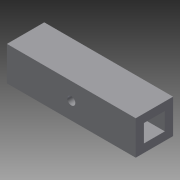
# Autodesk Inventor part: Truc Lumiere
Saved by Autodesk Inventor 2014 SP2 (Build 180246200, 246)
## iProperties
Created: 2014-11-04
Part Number: Truc Lumiere
Material: Générique
Document SubType Name: Modeling
Designer: sd
Density: 1 g/cm^3
Appearance: Par défaut
Author: sd
Autodesk Inventor part; units mm, degrees
ref_plane "YZ Plane" through (0, 0, 0) normal (1, 0, 0) x (0, 1, 0)
ref_plane "XZ Plane" through (0, 0, 0) normal (0, 1, 0) x (-1, 0, 0)
ref_plane "XY Plane" through (0, 0, 0) normal (0, 0, 1) x (1, 0, 0)
sketch "Esquisse1" plane through (0, 0, 0) normal (0, 1, 0) x (-1, 0, 0)
  line L0 (-20, 5.3) -> (20, 5.3)
  line L1 (20, 5.3) -> (20, -5.3)
  line L2 (20, -5.3) -> (-20, -5.3)
  line L3 (-20, -5.3) -> (-20, 5.3)
  point P0 (0, 0)
  dimension "d0" = 40
  dimension "d1" = 10.6
  dimension "d2" = 20
  dimension "d3" = 5.3
  constraints: 8 end point, 2 parallel, 1 horizontal, 1 perpendicular
  measures "d0" distance of L0.start L0.end
  measures "d1" distance of L2.end L0.start
  measures "d2" horizontal distance of point (0, 0) L0.start
  measures "d3" vertical distance of point (0, 0) L0.start
extrude "Extrusion1" add sketch "Esquisse1" along normal blind 11.6
sketch "Esquisse2" plane through (20, 0, 5.3) normal (1, 0, 0) x (0, 0, -1)
  line L0 (2.55, 9.05) -> (8.05, 9.05)
  line L1 (8.05, 9.05) -> (8.05, 2.55)
  line L2 (8.05, 2.55) -> (2.55, 2.55)
  line L3 (2.55, 2.55) -> (2.55, 9.05)
  point P0 (0, 11.6)
  point P1 (5.3, 0)
  dimension "d6" = 5.5
  dimension "d8" = 2.75
  dimension "d9" = 6.5
  dimension "d10" = 2.55
  constraints: 8 end point, 2 parallel, 1 horizontal, 1 perpendicular
  measures "d6" distance of L0.start L0.end
  measures "d8" horizontal distance of point (5.3, 0) L2.end
  measures "d9" distance of L2.end L0.start
  measures "d10" horizontal distance of point (0, 11.6) L0.start
extrude "Extrusion2" cut sketch "Esquisse2" against normal blind 8
sketch "Esquisse3" plane through (-20, 0, -5.3) normal (-1, 0, 0) x (0, 0, 1)
  line L0 (2.55, 9.05) -> (8.05, 9.05)
  line L1 (8.05, 9.05) -> (8.05, 2.55)
  line L2 (8.05, 2.55) -> (2.55, 2.55)
  line L3 (2.55, 2.55) -> (2.55, 9.05)
  point P0 (0, 11.6)
  point P1 (5.3, 0)
  dimension "d13" = 5.5
  dimension "d14" = 6.5
  dimension "d15" = 2.75
  dimension "d16" = 2.55
  constraints: 8 end point, 2 parallel, 1 horizontal, 1 perpendicular
  measures "d13" distance of L0.start L0.end
  measures "d14" distance of L2.end L0.start
  measures "d15" horizontal distance of point (5.3, 0) L0.start
  measures "d16" horizontal distance of point (0, 11.6) L0.start
extrude "Extrusion3" cut sketch "Esquisse3" against normal blind 8
sketch "Esquisse4" plane through (-12, 0, -5.3) normal (-1, 0, 0) x (0, 0, 1)
  line L0 (2.55, 9.05) -> (8.05, 9.05) projected
  line L1 (2.55, 2.55) -> (2.55, 9.05) projected
  circle A0 centre (5.3, 5.8) radius 1.25
  point P0 (5.3, 0)
  dimension "d19" = 2.5
  dimension "d20" = 3.25
  dimension "d21" = 2.75
  constraints: 1 centre point
  measures "d19" diameter of A0
  measures "d20" distance from line of L0 A0.centre
  measures "d21" distance from line of A0.centre L1
extrude "Extrusion4" cut sketch "Esquisse4" against normal through all
sketch "Esquisse5" plane through (0, 11.6, 0) normal (0, 1, 0) x (1, 0, 0)
  circle A0 centre (0, 0) radius 1.25
  dimension "d24" = 2.5
  constraints: 1 centre point, 1 coincident
  measures "d24" diameter of A0
extrude "Extrusion5" cut sketch "Esquisse5" against normal through all
equation "\"d2\" = 0.5 * d0"
equation "\"d3\" = 0.5 * d1"
equation "\"d8\" = 0.5 * d6"
equation "\"d10\" = -0.5 * d9 + 0.5 * d4"
equation "\"d15\" = 0.5 * d13"
equation "\"d16\" = -0.5 * d9 + 0.5 * d4"
equation "\"d20\" = 0.5 * d14"
equation "\"d4\" = 11.6"
